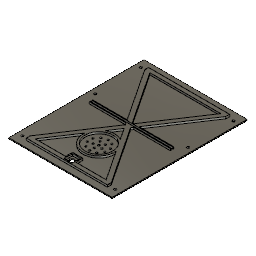
smmb_bottom (Autodesk Fusion 360 design; units mm, degrees)
Autodesk Fusion 360 part; units mm, degrees
sketch "Sketch1" plane through (0, 0, 0) normal (0, 0, 1) x (1, 0, 0)
  line L0 (0, 0) -> (134, 0)
  line L1 (134, 0) -> (134, 175.301)
  line L2 (134, 175.301) -> (0, 175.301)
  line L3 (0, 175.301) -> (0, 0)
  circle A0 centre (7, 164.301) radius 1.55
  circle A1 centre (7, 11) radius 1.55
  circle A2 centre (7, 105.301) radius 1.55
  line L4 (67, 0) -> (67, 175.301) construction
  circle A3 centre (127, 164.301) radius 1.55
  circle A4 centre (127, 105.301) radius 1.55
  circle A5 centre (127, 11) radius 1.55
  line L5 (0, 94.247) -> (134, 94.247)
  line L6 (0, 93.247) -> (134, 93.247)
  line L7 (0, 90.147) -> (134, 90.147)
  line L8 (0, 91.147) -> (134, 91.147)
  line L9 (7, 105.301) -> (7, 103.751)
  line L10 (14.5, 94.247) -> (14.5, 90.147)
  line L11 (7, 12.55) -> (7, 11)
  line L12 (127, 12.55) -> (127, 11)
  line L13 (127, 105.301) -> (127, 103.751)
  line L14 (119.5, 94.247) -> (119.5, 90.147)
  line L15 (7, 164.301) -> (127, 164.301) construction
  line L16 (7, 11) -> (127, 11) construction
  line L17 (119.5, 166.801) -> (14.5, 166.801)
  line L18 (14.5, 166.801) -> (14.5, 161.801)
  line L19 (14.5, 161.801) -> (119.5, 161.801)
  line L20 (119.5, 161.801) -> (119.5, 166.801)
  line L21 (119.5, 166.801) -> (14.5, 161.801) construction
  line L22 (14.5, 166.801) -> (119.5, 161.801) construction
  line L23 (119.5, 13.5) -> (14.5, 13.5)
  line L24 (14.5, 13.5) -> (14.5, 8.5)
  line L25 (14.5, 8.5) -> (119.5, 8.5)
  line L26 (119.5, 8.5) -> (119.5, 13.5)
  line L27 (119.5, 13.5) -> (14.5, 8.5) construction
  line L28 (14.5, 13.5) -> (119.5, 8.5) construction
  line L29 (14.5, 8.5) -> (119.5, 166.801)
  line L30 (119.5, 161.801) -> (17.8165, 8.5)
  line L31 (14.5, 13.5) -> (116.1835, 166.801)
  line L32 (14.5, 166.801) -> (119.5, 8.5)
  line L33 (119.5, 13.5) -> (17.8165, 166.801)
  line L34 (14.5, 161.801) -> (116.1835, 8.5)
  circle A6 centre (67, 50) radius 18
  circle A7 centre (67, 50) radius 20.5
  line L35 (67, 50) -> (42.7898, 13.5)
  line L36 (67, 50) -> (91.2102, 13.5)
  circle A8 centre (67, 50) radius 1.25
  circle A9 centre (67, 44) radius 1.25
  circle A10 centre (67, 38) radius 1.25
  circle A11 centre (72.7063, 48.1459) radius 1.25
  circle A12 centre (70.5267, 54.8541) radius 1.25
  circle A13 centre (63.4733, 54.8541) radius 1.25
  circle A14 centre (61.2937, 48.1459) radius 1.25
  circle A15 centre (74.0534, 40.2918) radius 1.25
  circle A16 centre (78.4127, 46.2918) radius 1.25
  circle A17 centre (78.4127, 53.7082) radius 1.25
  circle A18 centre (74.0534, 59.7082) radius 1.25
  circle A19 centre (67, 62) radius 1.25
  circle A20 centre (59.9466, 59.7082) radius 1.25
  circle A21 centre (55.5873, 53.7082) radius 1.25
  circle A22 centre (55.5873, 46.2918) radius 1.25
  circle A23 centre (59.9466, 40.2918) radius 1.25
  line L37 (72.1, 21) -> (61.9, 21)
  line L38 (61.9, 21) -> (61.9, 10)
  line L39 (61.9, 10) -> (72.1, 10)
  line L40 (72.1, 10) -> (72.1, 21)
  line L41 (72.1, 21) -> (61.9, 10) construction
  line L42 (61.9, 21) -> (72.1, 10) construction
  circle A24 centre (67, 15.5) radius 3
  line L43 (60.4, 22.5) -> (60.4, 8.5)
  line L44 (60.4, 8.5) -> (73.6, 8.5)
  line L45 (73.6, 8.5) -> (73.6, 22.5)
  line L46 (73.6, 22.5) -> (60.4, 22.5)
  line L47 (73.6, 22.5) -> (73.6, 30.5915)
  line L48 (60.4, 22.5) -> (60.4, 30.5915)
  point P0 (67, 164.301)
  point P1 (67, 11)
  point P2 (67, 15.5)
  dimension "d1" = 175.301
  dimension "d2" = 134
  dimension "d3" = 3.1
  dimension "d4" = 7
  dimension "d5" = 11
  dimension "d6" = 3.1
  dimension "d7" = 7
  dimension "d8" = 11
  dimension "d9" = 3.1
  dimension "d10" = 70
  dimension "d11" = 7
  dimension "d12" = 81.054
  dimension "d13" = 1
  dimension "d14" = 85.154
  dimension "d15" = -1
  dimension "d20" = 105
  dimension "d21" = 5
  dimension "d22" = 105
  dimension "d23" = 5
  dimension "d26" = 36
  dimension "d28" = 50
  dimension "d29" = 41
  dimension "d30" = 2.5
  dimension "d31" = 2.5
  dimension "d32" = 6
  dimension "d33" = 2.5
  dimension "d34" = 12
  dimension "d36" = 360
  dimension "d38" = 360
  dimension "d41" = 14.5
  dimension "d42" = 14.5
  dimension "d43" = 11
  dimension "d44" = 10.2
  dimension "d46" = 10
  dimension "d47" = 6
  dimension "d48" = 1.5
  constraint horizontal L0
  constraint vertical L1
  constraint horizontal L2
  constraint vertical L3
  constraint coincident L0.start L3.end
  constraint midpoint L0 L4.start
  constraint midpoint L2 L4.end
  constraint symmetric A0 L4 A3
  constraint symmetric A1 L4 A5
  constraint symmetric A2 L4 A4
  constraint coincident L3 L5.start
  constraint coincident L1 L5.end
  constraint perpendicular L1 L5
  constraint coincident L3 L7.start
  constraint coincident L1 L7.end
  constraint perpendicular L1 L7
  constraint coincident A2.centre L9.start
  constraint coincident A1.centre L11.end
  constraint perpendicular L8 L9
  constraint coincident A4.centre L13.start
  constraint coincident A5.centre L12.end
  constraint perpendicular L6 L13
  constraint coincident A2 L9.end
  constraint coincident L5 L10.start
  constraint coincident L7 L10.end
  constraint coincident A1 L11.start
  constraint coincident L7 L14.end
  constraint coincident A5 L12.start
  constraint collinear L12 L13
  constraint coincident A4 L13.end
  constraint coincident L5 L14.start
  constraint coincident A0.centre L15.start
  constraint coincident A3.centre L15.end
  constraint perpendicular L17 L18
  constraint parallel L17 L19
  constraint parallel L18 L20
  constraint horizontal L17
  constraint coincident L21 P0
  constraint coincident L22 P0
  constraint midpoint L15 P0
  constraint perpendicular L23 L24
  constraint parallel L23 L25
  constraint parallel L24 L26
  constraint horizontal L23
  constraint coincident L27 P1
  constraint coincident L28 P1
  constraint midpoint L16 P1
  constraint coincident L25 L30.end
  constraint parallel L29 L30
  constraint coincident L17 L31.end
  constraint parallel L30 L31
  constraint coincident L17 L33.end
  constraint parallel L32 L33
  constraint coincident L25 L34.end
  constraint parallel L33 L34
  constraint coincident L4 A6.centre
  constraint concentric A6 A7
  constraint coincident A6.centre A7.centre
  constraint coincident L23 L35.end
  constraint parallel L30 L35
  constraint coincident L23 L36.end
  constraint parallel L34 L36
  constraint concentric A7 A8
  constraint coincident L4 A9.centre
  constraint coincident L4 A10.centre
  constraint perpendicular L37 L38
  constraint parallel L37 L39
  constraint parallel L38 L40
  constraint horizontal L37
  constraint coincident L41 P2
  constraint coincident L42 P2
  constraint coincident L4 P2
  constraint coincident P2 A24.centre
  constraint coincident A7 L47.end
  constraint perpendicular L46 L47
  constraint coincident A7 L48.end
  constraint perpendicular L46 L48
  measures "d1" distance of L0.start L2.end
  measures "d2" distance of L0.start L0.end
  measures "d3" diameter of A0
  measures "d4" distance of L3 A0.centre
  measures "d5" distance of L2 A0.centre
  measures "d6" diameter of A1
  measures "d7" distance of L3 A1.centre
  measures "d8" distance of L0 A1.centre
  measures "d9" diameter of A2
  measures "d10" distance of L2 A2.centre
  measures "d11" distance of L3 A2.centre
  measures "d12" distance of L2 L5
  measures "d14" distance of L2 L7
  measures "d20" distance of L18.end L19.end
  measures "d21" distance of L17.end L18.end
  measures "d22" distance of L24.end L25.end
  measures "d23" distance of L23.end L24.end
  measures "d26" diameter of A6
  measures "d28" distance of L0 A6.centre
  measures "d29" diameter of A7
  measures "d30" diameter of A8
  measures "d31" diameter of A9
  measures "d32" distance of A6.centre A9.centre
  measures "d33" diameter of A10
  measures "d34" distance of A6.centre A10.centre
  measures "d41" distance of L3 L10
  measures "d42" distance of L1 L14
  measures "d43" distance of L37.end L38.end
  measures "d44" distance of L38.end L39.end
  measures "d46" distance of L0 L39
  measures "d47" diameter of A24
extrude "Extrude1" add sketch "Sketch1" along normal blind 1.5 contours L0 L1 L3 L7 L24 L25 L26 L30 L31 L33 L34 L44 | L3 L7 L8 L10 | L1 L7 L8 L14 | L3 L6 L8 L10 | L7 L8 L10 L34 | L1 L6 L8 L14 | L7 L8 L14 L30 | L3 L5 L6 L10 | L6 L8 L10 L34 | L7 L8 L32 L34 | L7 L31 L34 | L1 L5 L6 L14 | L6 L8 L14 L30 | L7 L30 L33 | L7 L8 L29 L30 | L1 L2 L3 L5 L17 L18 L20 L30 L34 | L5 L6 L10 L34 | L6 L8 L32 L34 | L7 L8 L31 L33 | L29 L31 L32 L34 | L8 L31 L32 | L7 L29 L32 | L23 L29 L31 L34 | L5 L6 L14 L30 | L6 L8 L29 L30 | L29 L30 L32 L33 | L8 L29 L33 | L23 L30 L32 L33 | L5 L6 L32 L34 | L6 L8 L31 L32 L33 | L8 L31 L33 | L29 L30 L32 L34 | L23 L24 L29 | L23 L29 L30 L34 A7 | L5 L6 L29 L30 | L6 L8 L29 L31 L33 | L23 L30 L32 L34 A7 | L23 L26 L32 | L5 L19 L32 L34 | L5 L6 L32 L33 | L6 L31 L33 | L23 L25 L29 L30 | L30 L34 A7 | L5 L19 L29 L30 | L5 L6 L29 L31 | L23 L25 L32 L34 | L5 L19 L32 L33 | L18 L19 L32 | L5 L6 L31 L33 | L23 L30 A7 L35 | L23 L25 L30 L43 | L30 L34 A6 A7 L35 L36 | L30 A7 | L34 A7 | L5 L19 L29 L31 | L19 L20 L29 | L23 L25 L34 L45 | L23 L34 A7 L36 | L5 L19 L31 L33 | L17 L19 L32 L33 | L23 A7 L35 L43 L48 | L23 L25 L38 L39 L40 L43 L44 L45 | L17 L19 L29 L31 | L23 A7 L36 L45 L47 | L17 L19 L31 L33 | L23 L37 L38 L40 L43 L45 L46 | A6 A7 L35 L36 | L23 L37 L38 L40 A24 | L23 L38 L39 L40 A24 | A7 L46 L47 L48 | A6 L35 L36 A8 A15 A23 | A6 L35 L36 A8 A15 A23 | L23 A24 | L23 A24 | L35 A23 | L35 A23 | L36 A15 | L36 A15 | L35 L36 A8 | L35 L36 A8 | A9 | A10 | A11 | A12 | A13 | A14 | A16 | A17 | A18 | A19 | A20 | A21 | A22
extrude "Extrude2" add sketch "Sketch1" along normal blind 4 contours L7 L8 L10 L34 | L7 L8 L14 L30 | L7 L8 L32 L34 | L7 L8 L29 L30 | L5 L6 L10 L34 | L7 L8 L31 L33 | L8 L31 L32 | L5 L6 L14 L30 | L8 L29 L33 | L5 L6 L32 L34 | L5 L6 L29 L30 | L5 L6 L32 L33 | L5 L6 L29 L31 | L5 L6 L31 L33
extrude "Extrude3" add sketch "Sketch1" along normal blind 4 contours L7 L31 L34 | L7 L30 L33 | L29 L31 L32 L34 | L7 L29 L32 | L23 L29 L31 L34 | L29 L30 L32 L33 | L23 L30 L32 L33 | L29 L30 L32 L34 | L23 L24 L29 | L23 L29 L30 L34 A7 | L23 L30 L32 L34 A7 | L23 L26 L32 | L5 L19 L32 L34 | L23 L25 L29 L30 | L5 L19 L29 L30 | L23 L25 L32 L34 | L5 L19 L32 L33 | L18 L19 L32 | L23 L25 L30 L43 | L30 L34 A6 A7 L35 L36 | L30 A7 | L34 A7 | L5 L19 L29 L31 | L19 L20 L29 | L23 L25 L34 L45 | L17 L19 L32 L33 | L23 L25 L38 L39 L40 L43 L44 L45 | L17 L19 L29 L31 | L17 L19 L31 L33 | L23 L37 L38 L40 L43 L45 L46 | A6 A7 L35 L36
extrude "Extrude4" cut sketch "Sketch1" along normal blind 1.5 contours L35 A23 | L35 A23 | L36 A15 | L36 A15 | L35 L36 A8 | L35 L36 A8 | A9 | A10 | A11 | A12 | A13 | A14 | A16 | A17 | A18 | A19 | A20 | A21 | A22
extrude "Extrude5" cut sketch "Sketch1" along normal blind 5 contours L23 A24 | L23 A24
equation "d6 = d3"
equation "d7 = d4"
equation "d8 = d5"
equation "d9 = d3"
equation "d11 = d4"
equation "d29 = d26 + 5 mm"
equation "d31 = d30"
equation "d32 = ( 36 / 2 / 3 ) * 1 mm"
equation "d33 = d30"
equation "d34 = d32 * 2"
equation "d42 = d41"
